Autodesk Fusion 360 part; units mm, degrees
note: some values were not read from the file. Chosen so that the rebuilt part matches the saved one: which bodies a step acts on; which face or edge a step refers to. Set by a fixed rule: which sketch regions a step uses.
(part 2 of 2)
sketch "Sketch24" plane through (0, 0, 25.4) normal (0, 0, 1) x (-1, 0, 0)
  line L0 (498.8821, -1295.4) -> (273.5385, -1295.4)
  line L1 (273.5385, -1295.4) -> (348.4359, -711.2)
  line L2 (348.4359, -711.2) -> (498.8821, -711.2)
  line L3 (498.8821, -711.2) -> (498.8821, -1295.4)
  line L4 (-12.7, -1879.6) -> (-228.6, -1879.6)
  line L5 (-228.6, -1879.6) -> (-228.6, -1701.8)
  line L6 (-228.6, -1701.8) -> (-12.7, -1701.8)
  line L7 (-12.7, -1701.8) -> (-12.7, -1879.6)
  line L8 (-279.4, -203.2) -> (-355.6, -203.2)
  line L9 (-355.6, -203.2) -> (-355.6, -25.4)
  line L10 (-355.6, -25.4) -> (-279.4, -25.4)
  line L11 (-279.4, -25.4) -> (-279.4, -203.2)
  line L12 (12.7, -1676.4) -> (12.7, -1473.2)
  line L13 (12.7, -1473.2) -> (228.6, -1473.2)
  line L14 (228.6, -1473.2) -> (228.6, -1676.4)
  line L15 (228.6, -1676.4) -> (12.7, -1676.4)
  line L16 (-165.1, -203.2) -> (-254, -203.2)
  line L17 (-254, -203.2) -> (-254, -25.4)
  line L18 (-254, -25.4) -> (-165.1, -25.4)
  line L19 (-165.1, -25.4) -> (-165.1, -203.2)
  line L20 (-355.6, -228.6) -> (-279.4, -228.6)
  line L21 (-279.4, -228.6) -> (-279.4, -355.6)
  line L22 (-279.4, -355.6) -> (-355.6, -355.6)
  line L23 (-355.6, -355.6) -> (-355.6, -228.6)
  line L24 (-12.7, -711.2) -> (-12.7, -1447.8)
  line L25 (-12.7, -1447.8) -> (-228.6, -1447.8)
  line L26 (-228.6, -1447.8) -> (-228.6, -1446.1784)
  line L27 (-228.6, -1446.1784) -> (-322.828, -711.2)
  line L28 (-322.828, -711.2) -> (-12.7, -711.2)
  line L29 (-139.7, -203.2) -> (-139.7, -25.4)
  line L30 (-139.7, -25.4) -> (355.6, -25.4)
  line L31 (355.6, -25.4) -> (355.6, -203.2)
  line L32 (355.6, -203.2) -> (-139.7, -203.2)
  line L33 (228.6, -1701.8) -> (228.6, -1879.6)
  line L34 (228.6, -1879.6) -> (12.7, -1879.6)
  line L35 (12.7, -1879.6) -> (12.7, -1701.8)
  line L36 (12.7, -1701.8) -> (228.6, -1701.8)
  line L37 (-355.6, -455.5784) -> (-355.3921, -457.2)
  line L38 (-355.3921, -457.2) -> (-12.7, -457.2)
  line L39 (-12.7, -457.2) -> (-12.7, -685.8)
  line L40 (-12.7, -685.8) -> (-326.0844, -685.8)
  line L41 (-326.0844, -685.8) -> (-355.3921, -457.2)
  line L42 (-355.3921, -457.2) -> (-355.6, -457.2)
  line L43 (-355.6, -457.2) -> (-355.6, -455.5784)
  line L44 (-12.7, -1676.4) -> (-228.6, -1676.4)
  line L45 (-228.6, -1676.4) -> (-228.6, -1473.2)
  line L46 (-228.6, -1473.2) -> (-12.7, -1473.2)
  line L47 (-12.7, -1473.2) -> (-12.7, -1676.4)
  line L48 (-165.1, -355.6) -> (-254, -355.6)
  line L49 (-254, -355.6) -> (-254, -228.6)
  line L50 (-254, -228.6) -> (-165.1, -228.6)
  line L51 (-165.1, -228.6) -> (-165.1, -355.6)
  line L52 (-355.6, -381) -> (355.6, -381)
  line L53 (355.6, -381) -> (355.6, -431.8)
  line L54 (355.6, -431.8) -> (-355.6, -431.8)
  line L55 (-355.6, -431.8) -> (-355.6, -381)
  line L56 (12.7, -685.8) -> (12.7, -457.2)
  line L57 (12.7, -457.2) -> (355.3921, -457.2)
  line L58 (355.3921, -457.2) -> (355.6, -455.5784)
  line L59 (355.6, -455.5784) -> (355.6, -457.2)
  line L60 (355.6, -457.2) -> (355.3921, -457.2)
  line L61 (355.3921, -457.2) -> (326.0844, -685.8)
  line L62 (326.0844, -685.8) -> (12.7, -685.8)
  line L63 (-139.7, -228.6) -> (355.6, -228.6)
  line L64 (355.6, -228.6) -> (355.6, -355.6)
  line L65 (355.6, -355.6) -> (-139.7, -355.6)
  line L66 (-139.7, -355.6) -> (-139.7, -228.6)
  line L67 (228.6, -1446.1784) -> (228.6, -1447.8)
  line L68 (228.6, -1447.8) -> (12.7, -1447.8)
  line L69 (12.7, -1447.8) -> (12.7, -711.2)
  line L70 (12.7, -711.2) -> (322.828, -711.2)
  line L71 (322.828, -711.2) -> (228.6, -1446.1784)
  line L72 (-273.5385, -1295.4) -> (-498.8821, -1295.4)
  line L73 (-498.8821, -1295.4) -> (-498.8821, -711.2)
  line L74 (-498.8821, -711.2) -> (-348.4359, -711.2)
  line L75 (-348.4359, -711.2) -> (-273.5385, -1295.4)
  line L76 (270.2821, -1320.8) -> (524.2821, -1320.8)
  line L77 (524.2821, -1320.8) -> (524.2821, -685.8)
  line L78 (524.2821, -685.8) -> (351.6923, -685.8)
  line L79 (351.6923, -685.8) -> (381, -457.2)
  line L80 (381, -457.2) -> (381, -228.6)
  line L81 (381, -228.6) -> (393.7, -228.6)
  line L82 (393.7, -228.6) -> (393.7, -203.2)
  line L83 (393.7, -203.2) -> (381, -203.2)
  line L84 (381, -203.2) -> (381, 0)
  line L85 (381, 0) -> (-381, 0)
  line L86 (-381, 0) -> (-381, -203.2)
  line L87 (-381, -203.2) -> (-508, -203.2)
  line L88 (-508, -203.2) -> (-508, -228.6)
  line L89 (-508, -228.6) -> (-381, -228.6)
  line L90 (-381, -228.6) -> (-381, -457.2)
  line L91 (-381, -457.2) -> (-351.6923, -685.8)
  line L92 (-351.6923, -685.8) -> (-524.2821, -685.8)
  line L93 (-524.2821, -685.8) -> (-524.2821, -1320.8)
  line L94 (-524.2821, -1320.8) -> (-270.2821, -1320.8)
  line L95 (-270.2821, -1320.8) -> (-254, -1447.8)
  line L96 (-254, -1447.8) -> (-254, -1676.4)
  line L97 (-254, -1676.4) -> (-393.7, -1676.4)
  line L98 (-393.7, -1676.4) -> (-393.7, -1701.8)
  line L99 (-393.7, -1701.8) -> (-254, -1701.8)
  line L100 (-254, -1701.8) -> (-254, -1905)
  line L101 (-254, -1905) -> (254, -1905)
  line L102 (254, -1905) -> (254, -1701.8)
  line L103 (254, -1701.8) -> (393.7, -1701.8)
  line L104 (393.7, -1701.8) -> (393.7, -1676.4)
  line L105 (393.7, -1676.4) -> (254, -1676.4)
  line L106 (254, -1676.4) -> (254, -1447.8)
  line L107 (254, -1447.8) -> (270.2821, -1320.8)
  line L108 (254, -1565.0031) -> (254, -1447.8)
  line L109 (381, -457.2) -> (355.6, -381)
  line L110 (355.6, -381) -> (355.6, -228.6)
  line L111 (254, -1447.8) -> (381, -457.2)
  line L112 (254, -1506.4016) -> (252.5, -1506.4016)
  line L113 (252.5, -1506.4016) -> (252.5, -1447.8)
  line L114 (252.5, -1447.8) -> (379.5, -457.2)
  line L115 (379.5, -457.2) -> (354.1, -381)
  line L116 (354.1, -381) -> (354.1, -228.6)
  line L117 (354.1, -228.6) -> (355.6, -228.6)
  point P0 (254, -1506.4016)
  dimension "d345" = 1.5
  constraint midpoint L108 P0
  constraint coincident L106 P0
  constraint coincident L106.end L107.start
  constraint coincident L79.end L80.start
  constraint coincident L52.end L53.start
  constraint coincident L63.end L64.start
  constraint coincident P0 L112.start
  constraint horizontal L112
  constraint perpendicular L112 L113
  constraint parallel L79 L114
  constraint coincident L52 L115.end
  constraint parallel L109 L115
  constraint coincident L63 L116.end
  constraint perpendicular L63 L116
  measures "d345" distance of P0 L112.end
sketch "Sketch25" plane through (-254, 0, 0) normal (-1, 0, 0) x (0, -1, 0)
  circle A0 centre (-1524, 12.78) radius 5
  line L0 (-1676.4, 0) -> (-1447.8, 0)
  line L1 (-1447.8, 0) -> (-1447.8, 25.4)
  line L2 (-1447.8, 25.4) -> (-1676.4, 25.4)
  line L3 (-1676.4, 25.4) -> (-1676.4, 0)
  line L4 (-1506.3949, 25.4) -> (-1506.3949, 26.9)
  line L5 (-1506.3949, 25.4) -> (-1507.3413, 26.3724)
  line L6 (-1507.3413, 26.3724) -> (-1530.641, 50.3126)
  line L7 (-1530.641, 50.3126) -> (-1530, 51)
  line L8 (-1506.3949, 26.9) -> (-1530, 51)
  constraint vertical L4
  constraint coincident L2 L4.start
  constraint parallel L5 L6
extrude "Extrude28" add sketch "Sketch25" against normal blind 1.5 contours L4 L5 L6 L7 L8 bodies 16 18 20 21 22 23 24 25
ref_plane "WorkPlane4" through (0, 482.6, 38.1) normal (0, -0.965926, -0.258819) x (1, 0, 0)
sketch "Sketch26" plane through (0, 459.7969, 123.2022) normal (0, -0.965926, -0.258819) x (1, 0, 0)
  line L0 (184.1911, -88.093) -> (-185, -88.093)
  line L1 (-185, -88.093) -> (-185, 419.907)
  line L2 (184.1911, -88.093) -> (184.1911, 419.907)
  arc A0 (-185, 419.907) -> (184.1911, 419.907) centre (-0.4045, 864.0338) ccw
  dimension "d352" = 508
  dimension "d353" = 508
  constraint horizontal L0
  constraint perpendicular L0 L1
  constraint perpendicular L0 L2
  measures "d352" distance of L0.end L1.end
  measures "d353" distance of L0.start L2.end
extrude "Extrude29" add sketch "Sketch26" along normal blind 12.7 separate body makes body 26
sketch "Sketch28" plane through (0, 0, 25.4) normal (0, 0, 1) x (-1, 0, 0)
  line L0 (498.8821, -1295.4) -> (273.5385, -1295.4)
  line L1 (273.5385, -1295.4) -> (348.4359, -711.2)
  line L2 (348.4359, -711.2) -> (498.8821, -711.2)
  line L3 (498.8821, -711.2) -> (498.8821, -1295.4)
  line L4 (-12.7, -1879.6) -> (-228.6, -1879.6)
  line L5 (-228.6, -1879.6) -> (-228.6, -1701.8)
  line L6 (-228.6, -1701.8) -> (-12.7, -1701.8)
  line L7 (-12.7, -1701.8) -> (-12.7, -1879.6)
  line L8 (-279.4, -203.2) -> (-355.6, -203.2)
  line L9 (-355.6, -203.2) -> (-355.6, -25.4)
  line L10 (-355.6, -25.4) -> (-279.4, -25.4)
  line L11 (-279.4, -25.4) -> (-279.4, -203.2)
  line L12 (12.7, -1676.4) -> (12.7, -1473.2)
  line L13 (12.7, -1473.2) -> (228.6, -1473.2)
  line L14 (228.6, -1473.2) -> (228.6, -1676.4)
  line L15 (228.6, -1676.4) -> (12.7, -1676.4)
  line L16 (-165.1, -203.2) -> (-254, -203.2)
  line L17 (-254, -203.2) -> (-254, -25.4)
  line L18 (-254, -25.4) -> (-165.1, -25.4)
  line L19 (-165.1, -25.4) -> (-165.1, -203.2)
  line L20 (-355.6, -228.6) -> (-279.4, -228.6)
  line L21 (-279.4, -228.6) -> (-279.4, -355.6)
  line L22 (-279.4, -355.6) -> (-355.6, -355.6)
  line L23 (-355.6, -355.6) -> (-355.6, -228.6)
  line L24 (-12.7, -711.2) -> (-12.7, -1447.8)
  line L25 (-12.7, -1447.8) -> (-228.6, -1447.8)
  line L26 (-228.6, -1447.8) -> (-228.6, -1446.1784)
  line L27 (-228.6, -1446.1784) -> (-322.828, -711.2)
  line L28 (-322.828, -711.2) -> (-12.7, -711.2)
  line L29 (-139.7, -203.2) -> (-139.7, -25.4)
  line L30 (-139.7, -25.4) -> (355.6, -25.4)
  line L31 (355.6, -25.4) -> (355.6, -203.2)
  line L32 (355.6, -203.2) -> (-139.7, -203.2)
  line L33 (228.6, -1701.8) -> (228.6, -1879.6)
  line L34 (228.6, -1879.6) -> (12.7, -1879.6)
  line L35 (12.7, -1879.6) -> (12.7, -1701.8)
  line L36 (12.7, -1701.8) -> (228.6, -1701.8)
  line L37 (-355.6, -455.5784) -> (-355.3921, -457.2)
  line L38 (-355.3921, -457.2) -> (-12.7, -457.2)
  line L39 (-12.7, -457.2) -> (-12.7, -685.8)
  line L40 (-12.7, -685.8) -> (-326.0844, -685.8)
  line L41 (-326.0844, -685.8) -> (-355.3921, -457.2)
  line L42 (-355.3921, -457.2) -> (-355.6, -457.2)
  line L43 (-355.6, -457.2) -> (-355.6, -455.5784)
  line L44 (-12.7, -1676.4) -> (-228.6, -1676.4)
  line L45 (-228.6, -1676.4) -> (-228.6, -1473.2)
  line L46 (-228.6, -1473.2) -> (-12.7, -1473.2)
  line L47 (-12.7, -1473.2) -> (-12.7, -1676.4)
  line L48 (-165.1, -355.6) -> (-254, -355.6)
  line L49 (-254, -355.6) -> (-254, -228.6)
  line L50 (-254, -228.6) -> (-165.1, -228.6)
  line L51 (-165.1, -228.6) -> (-165.1, -355.6)
  line L52 (-355.6, -381) -> (355.6, -381)
  line L53 (355.6, -381) -> (355.6, -431.8)
  line L54 (355.6, -431.8) -> (-355.6, -431.8)
  line L55 (-355.6, -431.8) -> (-355.6, -381)
  line L56 (12.7, -685.8) -> (12.7, -457.2)
  line L57 (12.7, -457.2) -> (355.3921, -457.2)
  line L58 (355.3921, -457.2) -> (355.6, -455.5784)
  line L59 (355.6, -455.5784) -> (355.6, -457.2)
  line L60 (355.6, -457.2) -> (355.3921, -457.2)
  line L61 (355.3921, -457.2) -> (326.0844, -685.8)
  line L62 (326.0844, -685.8) -> (12.7, -685.8)
  line L63 (-139.7, -228.6) -> (355.6, -228.6)
  line L64 (355.6, -228.6) -> (355.6, -355.6)
  line L65 (355.6, -355.6) -> (-139.7, -355.6)
  line L66 (-139.7, -355.6) -> (-139.7, -228.6)
  line L67 (228.6, -1446.1784) -> (228.6, -1447.8)
  line L68 (228.6, -1447.8) -> (12.7, -1447.8)
  line L69 (12.7, -1447.8) -> (12.7, -711.2)
  line L70 (12.7, -711.2) -> (322.828, -711.2)
  line L71 (322.828, -711.2) -> (228.6, -1446.1784)
  line L72 (-273.5385, -1295.4) -> (-498.8821, -1295.4)
  line L73 (-498.8821, -1295.4) -> (-498.8821, -711.2)
  line L74 (-498.8821, -711.2) -> (-348.4359, -711.2)
  line L75 (-348.4359, -711.2) -> (-273.5385, -1295.4)
  line L76 (270.2821, -1320.8) -> (524.2821, -1320.8)
  line L77 (524.2821, -1320.8) -> (524.2821, -685.8)
  line L78 (524.2821, -685.8) -> (351.6923, -685.8)
  line L79 (351.6923, -685.8) -> (381, -457.2)
  line L80 (381, -457.2) -> (381, -228.6)
  line L81 (381, -228.6) -> (393.7, -228.6)
  line L82 (393.7, -228.6) -> (393.7, -203.2)
  line L83 (393.7, -203.2) -> (381, -203.2)
  line L84 (381, -203.2) -> (381, 0)
  line L85 (381, 0) -> (-381, 0)
  line L86 (-381, 0) -> (-381, -203.2)
  line L87 (-381, -203.2) -> (-508, -203.2)
  line L88 (-508, -203.2) -> (-508, -228.6)
  line L89 (-508, -228.6) -> (-381, -228.6)
  line L90 (-381, -228.6) -> (-381, -457.2)
  line L91 (-381, -457.2) -> (-351.6923, -685.8)
  line L92 (-351.6923, -685.8) -> (-524.2821, -685.8)
  line L93 (-524.2821, -685.8) -> (-524.2821, -1320.8)
  line L94 (-524.2821, -1320.8) -> (-270.2821, -1320.8)
  line L95 (-270.2821, -1320.8) -> (-254, -1447.8)
  line L96 (-254, -1447.8) -> (-254, -1676.4)
  line L97 (-254, -1676.4) -> (-393.7, -1676.4)
  line L98 (-393.7, -1676.4) -> (-393.7, -1701.8)
  line L99 (-393.7, -1701.8) -> (-254, -1701.8)
  line L100 (-254, -1701.8) -> (-254, -1905)
  line L101 (-254, -1905) -> (254, -1905)
  line L102 (254, -1905) -> (254, -1701.8)
  line L103 (254, -1701.8) -> (393.7, -1701.8)
  line L104 (393.7, -1701.8) -> (393.7, -1676.4)
  line L105 (393.7, -1676.4) -> (254, -1676.4)
  line L106 (254, -1676.4) -> (254, -1506.3949)
  line L107 (254, -1506.3949) -> (254, -1447.8)
  line L108 (254, -1447.8) -> (270.2821, -1320.8)
  line L109 (381, -457.2) -> (355.6, -457.2)
  line L110 (355.6, -457.2) -> (355.6, -431.8)
  line L111 (355.6, -431.8) -> (381, -431.8)
  line L112 (381, -431.8) -> (381, -457.2)
  line L113 (-381, -457.2) -> (-355.6, -457.2)
  line L114 (-355.6, -457.2) -> (-355.6, -431.8)
  line L115 (-355.6, -431.8) -> (-381, -431.8)
  line L116 (-381, -431.8) -> (-381, -457.2)
  line L117 (270.2821, -1320.8) -> (244.8821, -1320.8)
  line L118 (273.5385, -1295.4) -> (248.1385, -1295.4)
  line L119 (270.2821, -1320.8) -> (273.5385, -1295.4)
  line L120 (244.8821, -1320.8) -> (248.1385, -1295.4)
  line L121 (-270.2821, -1320.8) -> (-273.512, -1295.6062)
  line L122 (-273.512, -1295.6062) -> (-248.112, -1295.6062)
  line L123 (-248.112, -1295.6062) -> (-244.8821, -1320.8)
  line L124 (-244.8821, -1320.8) -> (-270.2821, -1320.8)
  line L125 (355.6, -431.8) -> (355.6, -1295.4)
  line L126 (381, -457.2) -> (381, -1295.4)
  line L127 (355.6, -1295.4) -> (381, -1295.4)
  line L128 (381, -1295.4) -> (381, -1320.8)
  line L129 (355.6, -1295.4) -> (355.6, -1320.8)
  line L130 (355.6, -1320.8) -> (381, -1320.8)
  line L131 (-355.6, -431.8) -> (-355.6, -1295.4)
  line L132 (-381, -457.2) -> (-381, -1295.4)
  line L133 (-381, -1295.4) -> (-355.6, -1295.4)
  line L134 (-355.6, -1295.4) -> (-355.6, -1320.8)
  line L135 (-381, -1295.4) -> (-381, -1320.8)
  line L136 (-381, -1320.8) -> (-355.6, -1320.8)
  line L137 (254, -1506.3949) -> (252.5, -1506.3949)
  line L138 (252.5, -1506.3949) -> (254, -1506.3949)
  dimension "d362" = 25.4
  dimension "d363" = 25.4
  dimension "d364" = 25.4
  dimension "d365" = 25.4
  dimension "d366" = 25.4
  constraint horizontal L109
  constraint vertical L110
  constraint horizontal L111
  constraint vertical L112
  constraint coincident L53.end L54.start
  constraint coincident L79.end L80.start
  constraint horizontal L113
  constraint vertical L114
  constraint horizontal L115
  constraint vertical L116
  constraint coincident L54.end L55.start
  constraint coincident L90.end L91.start
  constraint coincident L76.start L108.end
  constraint parallel L76 L117
  constraint coincident L0.end L1.start
  constraint parallel L0 L118
  constraint coincident L94.end L95.start
  constraint parallel L75 L121
  constraint parallel L72 L122
  constraint parallel L94 L124
  constraint coincident L0 L125.end
  constraint perpendicular L0 L125
  constraint coincident L0 L126.end
  constraint perpendicular L0 L126
  constraint coincident L76 L128.end
  constraint perpendicular L76 L128
  constraint coincident L76 L129.end
  constraint perpendicular L76 L129
  constraint coincident L72 L131.end
  constraint perpendicular L72 L131
  constraint coincident L72 L132.end
  constraint perpendicular L72 L132
  constraint coincident L94 L134.end
  constraint perpendicular L94 L134
  constraint coincident L94 L135.end
  constraint perpendicular L94 L135
  measures "d362" distance of L76.start L117.end
  measures "d363" distance of L0.end L118.end
  measures "d364" distance of L94.end L123.end
  measures "d365" distance of L94.end L121.end
  measures "d366" distance of L121.end L122.end
extrude "Extrude32" add sketch "Sketch28" along normal blind 152.4 separate body contours L0 L76 L127 L128 L129 L130 | L59 L80 L109 L110 L111 L112 L125 | L43 L90 L113 L114 L115 L116 L131 | L72 L94 L133 L134 L135 L136 makes body 27 at (-364.0667, 1320.8, 127) makes body 28 at (-364.0667, 431.8, 76.2) makes body 29 at (364.0667, 1295.4, 76.2) makes body 30 at (372.5333, 457.2, 127)
sketch "Sketch29" plane through (0, 0, 177.8) normal (0, 0, 1) x (-1, 0, 0)
  line L0 (381, -431.8) -> (355.6, -431.8)
  line L1 (355.6, -431.8) -> (355.6, -457.2)
  line L2 (355.6, -457.2) -> (381, -457.2)
  line L3 (381, -457.2) -> (381, -431.8)
  line L4 (381, -457.2) -> (355.6, -457.2)
  line L5 (355.6, -457.2) -> (355.6, -431.8)
  line L6 (355.6, -431.8) -> (381, -431.8)
  line L7 (381, -431.8) -> (381, -457.2)
  line L8 (-355.6, -431.8) -> (-381, -431.8)
  line L9 (-381, -431.8) -> (-381, -457.2)
  line L10 (-381, -457.2) -> (-355.6, -457.2)
  line L11 (-355.6, -457.2) -> (-355.6, -431.8)
  line L12 (381, -457.2) -> (270.3, -1320.8)
  line L13 (270.3, -1320.8) -> (245, -1320.8)
  line L14 (245, -1320.8) -> (355.6, -457.2)
  line L15 (-381, -457.2) -> (-270.3, -1320.8)
  line L16 (-270.3, -1320.8) -> (-244.9, -1320.8)
  line L17 (-244.9, -1320.8) -> (-355.6, -457.2)
  constraint horizontal L4
  constraint vertical L5
  constraint horizontal L6
  constraint vertical L7
  constraint coincident L0.end L1.start
  constraint coincident L2.end L3.start
  constraint horizontal L8
  constraint vertical L9
  constraint horizontal L10
  constraint vertical L11
  constraint perpendicular L3 L13
  constraint coincident L1.end L2.start
  constraint perpendicular L9 L16
sketch "Sketch30" plane through (0, 1136.8154, 796.0067) normal (0, 0.819152, 0.573576) x (-1, 0, 0)
  line L0 (12.7169, -880.4638) -> (12.7169, -537.5638)
  line L1 (12.7169, -537.5638) -> (12.7169, -512.1638)
  line L2 (12.7169, -512.1638) -> (-12.6831, -512.1638)
  line L3 (-12.6831, -512.1638) -> (-12.6831, -537.5638)
  line L4 (-12.6831, -537.5638) -> (-12.6831, -880.4638)
  line L5 (-12.6831, -880.4638) -> (12.7169, -880.4638)
split "Split3" by plane through (0, 308.3339, -440.3465) normal (0, 0.573576, -0.819152) bodies 19 makes body 31 at (-12.7169, 1562.3979, 158.6895)
sketch "Sketch31" plane through (0, 308.3339, -440.3465) normal (0, -0.573576, 0.819152) x (1, 0, 0)
  line L0 (12.6831, 1387.7953) -> (-12.7169, 1387.7953)
  line L1 (-12.7169, 1387.7953) -> (-12.7169, 1362.3953)
  line L2 (-12.7169, 1362.3953) -> (12.6831, 1362.3953)
  line L3 (12.6831, 1362.3953) -> (12.6831, 1387.7953)
  circle A0 centre (-0.0169, 1375.0953) radius 9.525
  point P0 (-0.0169, 1375.0953)
  dimension "d371" = 12.7
  dimension "d372" = 12.7
  dimension "d373" = 19.05
  constraint coincident P0 A0.centre
  measures "d371" distance of L3 P0
  measures "d372" distance of L2 P0
  measures "d373" diameter of A0
extrude "Extrude34" add sketch "Sketch31" against normal blind 350 contours A0 bodies 18
delete_body "RemoveBody1" bodies 31
sketch "Sketch32" plane through (0, 0, 25.4) normal (0, 0, 1) x (-1, 0, 0)
  line L0 (498.8821, -1295.4) -> (273.5385, -1295.4)
  line L1 (273.5385, -1295.4) -> (348.4359, -711.2)
  line L2 (348.4359, -711.2) -> (498.8821, -711.2)
  line L3 (498.8821, -711.2) -> (498.8821, -1295.4)
  line L4 (-12.7, -1879.6) -> (-228.6, -1879.6)
  line L5 (-228.6, -1879.6) -> (-228.6, -1701.8)
  line L6 (-228.6, -1701.8) -> (-12.7, -1701.8)
  line L7 (-12.7, -1701.8) -> (-12.7, -1879.6)
  line L8 (-279.4, -203.2) -> (-355.6, -203.2)
  line L9 (-355.6, -203.2) -> (-355.6, -25.4)
  line L10 (-355.6, -25.4) -> (-279.4, -25.4)
  line L11 (-279.4, -25.4) -> (-279.4, -203.2)
  line L12 (12.7, -1676.4) -> (12.7, -1473.2)
  line L13 (12.7, -1473.2) -> (228.6, -1473.2)
  line L14 (228.6, -1473.2) -> (228.6, -1676.4)
  line L15 (228.6, -1676.4) -> (12.7, -1676.4)
  line L16 (-165.1, -203.2) -> (-254, -203.2)
  line L17 (-254, -203.2) -> (-254, -25.4)
  line L18 (-254, -25.4) -> (-165.1, -25.4)
  line L19 (-165.1, -25.4) -> (-165.1, -203.2)
  line L20 (-355.6, -228.6) -> (-279.4, -228.6)
  line L21 (-279.4, -228.6) -> (-279.4, -355.6)
  line L22 (-279.4, -355.6) -> (-355.6, -355.6)
  line L23 (-355.6, -355.6) -> (-355.6, -228.6)
  line L24 (-12.7, -711.2) -> (-12.7, -1447.8)
  line L25 (-12.7, -1447.8) -> (-228.6, -1447.8)
  line L26 (-228.6, -1447.8) -> (-228.6, -1446.1784)
  line L27 (-228.6, -1446.1784) -> (-322.828, -711.2)
  line L28 (-322.828, -711.2) -> (-12.7, -711.2)
  line L29 (-139.7, -203.2) -> (-139.7, -25.4)
  line L30 (-139.7, -25.4) -> (355.6, -25.4)
  line L31 (355.6, -25.4) -> (355.6, -203.2)
  line L32 (355.6, -203.2) -> (-139.7, -203.2)
  line L33 (228.6, -1701.8) -> (228.6, -1879.6)
  line L34 (228.6, -1879.6) -> (12.7, -1879.6)
  line L35 (12.7, -1879.6) -> (12.7, -1701.8)
  line L36 (12.7, -1701.8) -> (228.6, -1701.8)
  line L37 (-355.6, -455.5784) -> (-355.3921, -457.2)
  line L38 (-355.3921, -457.2) -> (-12.7, -457.2)
  line L39 (-12.7, -457.2) -> (-12.7, -685.8)
  line L40 (-12.7, -685.8) -> (-326.0844, -685.8)
  line L41 (-326.0844, -685.8) -> (-355.3921, -457.2)
  line L42 (-355.3921, -457.2) -> (-355.6, -457.2)
  line L43 (-355.6, -457.2) -> (-355.6, -455.5784)
  line L44 (-12.7, -1676.4) -> (-228.6, -1676.4)
  line L45 (-228.6, -1676.4) -> (-228.6, -1473.2)
  line L46 (-228.6, -1473.2) -> (-12.7, -1473.2)
  line L47 (-12.7, -1473.2) -> (-12.7, -1676.4)
  line L48 (-165.1, -355.6) -> (-254, -355.6)
  line L49 (-254, -355.6) -> (-254, -228.6)
  line L50 (-254, -228.6) -> (-165.1, -228.6)
  line L51 (-165.1, -228.6) -> (-165.1, -355.6)
  line L52 (-355.6, -381) -> (355.6, -381)
  line L53 (355.6, -381) -> (355.6, -431.8)
  line L54 (355.6, -431.8) -> (-355.6, -431.8)
  line L55 (-355.6, -431.8) -> (-355.6, -381)
  line L56 (12.7, -685.8) -> (12.7, -457.2)
  line L57 (12.7, -457.2) -> (355.3921, -457.2)
  line L58 (355.3921, -457.2) -> (355.6, -455.5784)
  line L59 (355.6, -455.5784) -> (355.6, -457.2)
  line L60 (355.6, -457.2) -> (355.3921, -457.2)
  line L61 (355.3921, -457.2) -> (326.0844, -685.8)
  line L62 (326.0844, -685.8) -> (12.7, -685.8)
  line L63 (-139.7, -228.6) -> (355.6, -228.6)
  line L64 (355.6, -228.6) -> (355.6, -355.6)
  line L65 (355.6, -355.6) -> (-139.7, -355.6)
  line L66 (-139.7, -355.6) -> (-139.7, -228.6)
  line L67 (228.6, -1446.1784) -> (228.6, -1447.8)
  line L68 (228.6, -1447.8) -> (12.7, -1447.8)
  line L69 (12.7, -1447.8) -> (12.7, -711.2)
  line L70 (12.7, -711.2) -> (322.828, -711.2)
  line L71 (322.828, -711.2) -> (228.6, -1446.1784)
  line L72 (-273.5385, -1295.4) -> (-498.8821, -1295.4)
  line L73 (-498.8821, -1295.4) -> (-498.8821, -711.2)
  line L74 (-498.8821, -711.2) -> (-348.4359, -711.2)
  line L75 (-348.4359, -711.2) -> (-273.5385, -1295.4)
  line L76 (270.2821, -1320.8) -> (524.2821, -1320.8)
  line L77 (524.2821, -1320.8) -> (524.2821, -685.8)
  line L78 (524.2821, -685.8) -> (351.6923, -685.8)
  line L79 (351.6923, -685.8) -> (381, -457.2)
  line L80 (381, -457.2) -> (381, -228.6)
  line L81 (381, -228.6) -> (393.7, -228.6)
  line L82 (393.7, -228.6) -> (393.7, -203.2)
  line L83 (393.7, -203.2) -> (381, -203.2)
  line L84 (381, -203.2) -> (381, 0)
  line L85 (381, 0) -> (-381, 0)
  line L86 (-381, 0) -> (-381, -203.2)
  line L87 (-381, -203.2) -> (-508, -203.2)
  line L88 (-508, -203.2) -> (-508, -228.6)
  line L89 (-508, -228.6) -> (-381, -228.6)
  line L90 (-381, -228.6) -> (-381, -457.2)
  line L91 (-381, -457.2) -> (-351.6923, -685.8)
  line L92 (-351.6923, -685.8) -> (-524.2821, -685.8)
  line L93 (-524.2821, -685.8) -> (-524.2821, -1320.8)
  line L94 (-524.2821, -1320.8) -> (-270.2821, -1320.8)
  line L95 (-270.2821, -1320.8) -> (-254, -1447.8)
  line L96 (-254, -1447.8) -> (-254, -1676.4)
  line L97 (-254, -1676.4) -> (-393.7, -1676.4)
  line L98 (-393.7, -1676.4) -> (-393.7, -1701.8)
  line L99 (-393.7, -1701.8) -> (-254, -1701.8)
  line L100 (-254, -1701.8) -> (-254, -1905)
  line L101 (-254, -1905) -> (254, -1905)
  line L102 (254, -1905) -> (254, -1701.8)
  line L103 (254, -1701.8) -> (393.7, -1701.8)
  line L104 (393.7, -1701.8) -> (393.7, -1676.4)
  line L105 (393.7, -1676.4) -> (254, -1676.4)
  line L106 (254, -1676.4) -> (254, -1506.3949)
  line L107 (254, -1506.3949) -> (254, -1447.8)
  line L108 (254, -1447.8) -> (270.2821, -1320.8)
  circle A0 centre (0, -1460.5) radius 7.9375
  line L109 (-12.7, -1447.8) -> (-12.7, -1473.2)
  line L110 (12.7, -1447.8) -> (-12.7, -1447.8)
  line L111 (254, -1506.3949) -> (252.5, -1506.3949)
  line L112 (252.5, -1506.3949) -> (254, -1506.3949)
  dimension "d377" = 15.875
  dimension "d403" = 12.7
  dimension "d404" = 12.7
  constraint coincident L24.end L25.start
  constraint coincident L46.end L47.start
  constraint coincident L68.end L69.start
  measures "d377" diameter of A0
  measures "d403" distance of A0.centre L109
  measures "d404" distance of A0.centre L110
extrude "Extrude36" add sketch "Sketch32" along normal blind 290 separate body contours A0 makes body 32
sketch "Sketch33" plane through (-552.45, 0, 0) normal (-1, 0, 0) x (0, -1, 0)
  circle A0 centre (-1689.1, 30) radius 7.9375
  circle A1 centre (-1689.1, 30) radius 177.8
  dimension "d383" = 355.6
  constraint concentric A0 A1
  measures "d383" diameter of A1
sketch "Sketch34" plane through (552.45, 0, 0) normal (1, 0, 0) x (0, 1, 0)
  circle A0 centre (1689.1, 30) radius 7.9375
  circle A1 centre (1689.1, 30) radius 177.8
  dimension "d384" = 355.6
  constraint concentric A0 A1
  measures "d384" diameter of A1
sketch "Sketch35" plane through (-508, 0, 0) normal (-1, 0, 0) x (0, -1, 0)
  line L0 (-228.6, 0) -> (-203.2, 0)
  line L1 (-203.2, 0) -> (-203.2, 25.4)
  line L2 (-203.2, 25.4) -> (-228.6, 25.4)
  line L3 (-228.6, 25.4) -> (-228.6, 0)
  circle A0 centre (-215.9, 12.7) radius 184.15
  point P0 (-215.9, 12.7)
  dimension "d385" = 12.7
  dimension "d386" = 12.7
  dimension "d387" = 368.3
  constraint coincident P0 A0.centre
  measures "d385" distance of L1 P0
  measures "d386" distance of L0 P0
  measures "d387" diameter of A0
sketch "Sketch36" plane through (508, 0, 0) normal (1, 0, 0) x (0, 1, 0)
  line L0 (203.2, 0) -> (228.6, 0)
  line L1 (228.6, 0) -> (228.6, 25.4)
  line L2 (228.6, 25.4) -> (203.2, 25.4)
  line L3 (203.2, 25.4) -> (203.2, 0)
  circle A0 centre (215.9, 12.7) radius 184.15
  point P0 (215.9, 12.7)
  dimension "d388" = 12.7
  dimension "d389" = 12.7
  dimension "d390" = 368.3
  constraint coincident P0 A0.centre
  measures "d388" distance of L2 P0
  measures "d389" distance of L3 P0
  measures "d390" diameter of A0
extrude "Extrude37" add sketch "Sketch33" along normal blind 33.02 and the other way blind 101.6 separate body contours A0 | A1 makes body 33
extrude "Extrude38" add sketch "Sketch34" along normal blind 33.02 and the other way blind 101.6 separate body contours A0 | A1 makes body 34
extrude "Extrude39" add sketch "Sketch35" along normal mid plane 139.7 separate body contours L0 L1 L2 L3 | A0 makes body 35
extrude "Extrude40" add sketch "Sketch36" along normal mid plane 139.7 separate body contours L0 L1 L2 L3 | A0 makes body 36
ref_plane "WorkPlane5" through (120.65, 1447.8, 25.4) normal (0, -1, 0) x (1, 0, 0)
sketch "Sketch37" plane through (0, 1447.8, 0) normal (0, -1, 0) x (-1, 0, 0)
  line L0 (12.6175, -0.3683) -> (-12.6055, -0.3683)
  line L1 (-12.6055, -0.3683) -> (-12.6055, -392.2)
  line L2 (-12.6055, -392.2) -> (12.6175, -392.2)
  line L3 (12.6175, -392.2) -> (12.6175, -0.3683)
  point P0 (2.4262, -339.9473)
  constraint horizontal L0
  constraint vertical L1
  constraint horizontal L2
  constraint vertical L3
extrude "Extrude41" cut sketch "Sketch37" along normal blind 25 bodies 16 18
sketch "Sketch38" plane through (0, 1447.8, 0) normal (0, -1, 0) x (1, 0, 0)
  ellipse E0 centre (-0.0169, 329.7329) end of major axis (-0.0169, 313.1265) minor radius 9.525
  line L0 (-15, 350) -> (15, 350)
  line L1 (15, 350) -> (15, 310)
  line L2 (15, 310) -> (-15, 310)
  line L3 (-15, 310) -> (-15, 350)
  circle A0 centre (-0.0169, 329.7329) radius 9.525
  dimension "d412" = 19.05
  constraint horizontal L0
  constraint vertical L1
  constraint horizontal L2
  constraint vertical L3
  constraint concentric E0 A0
  measures "d412" diameter of A0
extrude "Extrude42" add sketch "Sketch38" along normal blind 50.8 separate body makes body 37
extrude "Extrude43" add 1 faces at (3.1216, 1447.8, 332.256) along direction (0, -1, 0) blind 177.8 on bodies 18 bodies 18 37
chamfer "Chamfer2" distance 5 angle 45 4 edges at (15, 1422.4, 350) (15, 1422.4, 310) (-15, 1422.4, 350) (-15, 1422.4, 310) on bodies 18
extrude "Extrude44" add sketch "Sketch28" along normal blind 25.4 from surface at 152.4 separate body contours L0 L76 L127 L128 L129 L130 | L0 L2 L125 L126 L127 | L2 L78 L125 L126 | L78 L79 L125 L126 | L59 L80 L109 L110 L111 L112 L125 | L79 L109 L125 | L43 L90 L113 L114 L115 L116 L131 | L91 L113 L131 | L91 L92 L131 L132 | L74 L92 L131 L132 | L72 L74 L131 L132 L133 | L72 L94 L133 L134 L135 L136 makes body 38 at (372.5333, 728.1333, 177.8) makes body 39 at (-372.5333, 728.1333, 177.8)
hidden bodies 19 33 34 35 36
